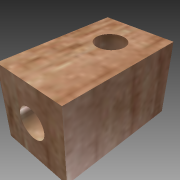
# Autodesk Inventor part: Top_RodHolder
Saved by Autodesk Inventor 2014 (Build 180170000, 170)
## iProperties
Created: 2013-12-11
Part Number: Top_RodHolder
Material: Birch
Document SubType Name: Modeling
Designer: Bram
Density: 0.512 g/cm^3
Appearance: Birch - Natural Medium Gloss
Author: Bram
Autodesk Inventor part; units mm, degrees
ref_plane "YZ Plane" through (0, 0, 0) normal (1, 0, 0) x (0, 1, 0)
ref_plane "XZ Plane" through (0, 0, 0) normal (0, 1, 0) x (-1, 0, 0)
ref_plane "XY Plane" through (0, 0, 0) normal (0, 0, 1) x (1, 0, 0)
sketch "Sketch1" plane through (0, 0, 0) normal (0, 0, 1) x (1, 0, 0)
  line L0 (0, 0) -> (20, 0)
  line L1 (20, 0) -> (20, 33)
  line L2 (20, 33) -> (0, 33)
  line L3 (0, 33) -> (0, 0)
  line L4 (6, 15) -> (6, 0)
  line L5 (14, 15) -> (14, 0)
  line L6 (6, 15) -> (14, 15)
  line L7 (10, 0) -> (10, 23)
  circle A0 centre (10, 23) radius 4
  dimension "d5" = 23
  dimension "d6" = 8
  constraints: 16 end point, 5 perpendicular, 2 parallel, 2 point on line, 1 centre point, 1 coincident, 1 horizontal, 1 midpoint
  measures "d5" distance of L7.start L7.end
  measures "d6" diameter of A0
extrude "Extrusion1" add sketch "Sketch1" along normal blind 20
sketch "Sketch2" plane through (0, 0, 0) normal (0, -1, 0) x (1, 0, 0)
  circle A0 centre (10, 10) radius 4
  dimension "d9" = 8
  constraints: 1 centre point
  measures "d9" diameter of A0
extrude "Extrusion2" cut sketch "Sketch2" against normal blind 15
body "Solid1"
